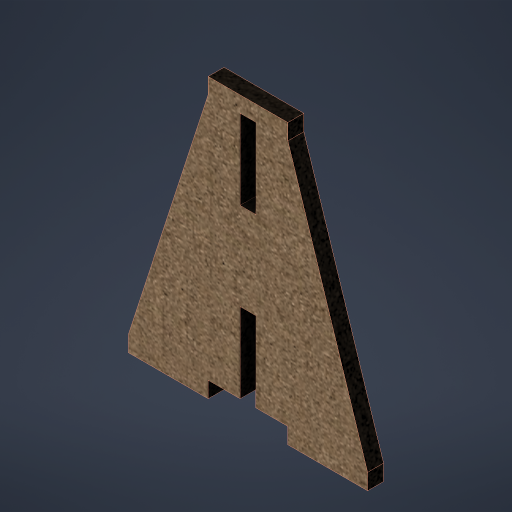
# Autodesk Inventor part: LightGate_Plate
Saved by Autodesk Inventor 2024.1 (Build 281209000, 209)
## iProperties
Created: 2023-05-21
Part Number: LightGate_Plate
Material: MDF Medium Density Fiberboard
Document SubType Name: Modeling
Designer: jaege
Density: 0.8 g/cm^3
Appearance: Red Oak - Natural Low Gloss
Author: jaege
Autodesk Inventor part; units mm, degrees
ref_plane "YZ Plane" through (0, 0, 0) normal (1, 0, 0) x (0, 1, 0)
ref_plane "XZ Plane" through (0, 0, 0) normal (0, 1, 0) x (-1, 0, 0)
ref_plane "XY Plane" through (0, 0, 0) normal (0, 0, 1) x (1, 0, 0)
sketch "Sketch1" plane through (0, 0, 0) normal (0, 0, 1) x (1, 0, 0)
  line L0 (-30, -35) -> (-10, -35)
  line L1 (-10, -35) -> (-10, -31)
  line L2 (-10, -31) -> (10, -31)
  line L3 (10, -31) -> (10, -35)
  line L4 (10, -35) -> (30, -35)
  line L5 (30, -35) -> (30, -31)
  line L6 (10, 35) -> (-10, 35)
  line L7 (-30, -31) -> (-30, -35)
  line L8 (-10, 35) -> (-10, 31)
  line L9 (-10, 31) -> (-30, -31)
  line L10 (10, 35) -> (10, 31)
  line L11 (10, 31) -> (30, -31)
  line L12 (-2, 31) -> (2, 31)
  line L13 (2, 31) -> (2, 11)
  line L14 (2, 11) -> (-2, 11)
  line L15 (-2, 11) -> (-2, 31)
  line L16 (2, -11) -> (-2, -11)
  line L17 (-2, -11) -> (-2, -31)
  line L18 (-2, -31) -> (2, -31)
  line L19 (2, -31) -> (2, -11)
  line L20 (0, 31) -> (0, -31) construction
  point P0 (0, 0)
  point P1 (0, 0)
  point P2 (-2, -31)
  point P3 (2, -31)
  dimension "d0" = 4
  dimension "d1" = 20
  dimension "d2" = 20
  dimension "d3" = 20
  dimension "d4" = 20
  dimension "d5" = 4
  dimension "d6" = 4
  dimension "d7" = 62
  dimension "d8" = 20
  dimension "d9" = 20
  dimension "d10" = 4
  constraints: 42 end point, 7 perpendicular, 6 parallel, 3 collinear, 3 horizontal, 3 horizontal alignment, 3 midpoint, 3 point on line, 2 coincident, 1 equal length, 1 vertical, 1 other
  measures "d0" distance of L7.start L0.start
  measures "d1" distance of L0.start L0.end
  measures "d2" distance of L3.end L4.end
  measures "d3" distance of L1.end L2.end
  measures "d4" distance of L6.start L6.end
  measures "d5" distance of L6.end L8.end
  measures "d6" distance of L6.start L10.end
  measures "d7" distance from line of L2 L10.end
  measures "d8" distance of L14.end L12.start
  measures "d9" distance of L16.end L17.end
  measures "d10" distance of L12.start L12.end
extrude "Extrusion1" add sketch "Sketch1" along normal blind 4 contours L7 L9 L8 L6 L10 L11 L5 L4 L3 L2 L19 L16 L17 L1 L0
body "Solid1"
